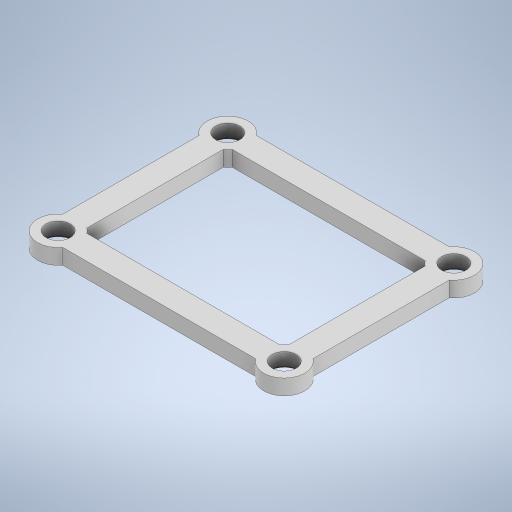
# Autodesk Inventor part: BasePlate
Saved by Autodesk Inventor 2024.2 (Build 282272000, 272)
## iProperties
Created: 2024-04-02
Part Number: BasePlate
Material: Generic
Document SubType Name: Modeling
Designer: ringl
Density: 1 g/cm^3
Appearance: Default
Author: ringl
Autodesk Inventor part; units mm, degrees
ref_plane "YZ Plane" through (0, 0, 0) normal (1, 0, 0) x (0, 1, 0)
ref_plane "XZ Plane" through (0, 0, 0) normal (0, 1, 0) x (-1, 0, 0)
ref_plane "XY Plane" through (0, 0, 0) normal (0, 0, 1) x (1, 0, 0)
sketch "Sketch1" plane through (0, 0, 0) normal (0, 1, 0) x (-1, 0, 0)
  circle A0 centre (0, 0) radius 2.35
  circle A1 centre (-44, 0) radius 2.35
  circle A2 centre (0, 33) radius 2.35
  circle A3 centre (-44, 33) radius 2.35
  line L0 (-3.2369, 30.65) -> (-40.7631, 30.65)
  line L1 (-40.7631, 35.35) -> (-3.2369, 35.35)
  line L2 (2.35, 29.7631) -> (2.35, 3.2369)
  line L3 (-2.35, 3.2369) -> (-2.35, 29.7631)
  line L4 (-3.2369, -2.35) -> (-40.7631, -2.35)
  line L5 (-40.7631, 2.35) -> (-3.2369, 2.35)
  arc A4 (-3.2369, -2.35) -> (2.35, 3.2369) centre (0, 0) ccw
  arc A5 (-2.35, 3.2369) -> (-3.2369, 2.35) centre (0, 0) ccw
  arc A6 (2.35, 29.7631) -> (-3.2369, 35.35) centre (0, 33) ccw
  arc A7 (-3.2369, 30.65) -> (-2.35, 29.7631) centre (0, 33) ccw
  line L6 (-41.65, 3.2369) -> (-41.65, 29.7631)
  line L7 (-46.35, 29.7631) -> (-46.35, 3.2369)
  arc A8 (-40.7631, 35.35) -> (-46.35, 29.7631) centre (-44, 33) ccw
  arc A9 (-41.65, 29.7631) -> (-40.7631, 30.65) centre (-44, 33) ccw
  arc A10 (-46.35, 3.2369) -> (-40.7631, -2.35) centre (-44, 0) ccw
  arc A11 (-40.7631, 2.35) -> (-41.65, 3.2369) centre (-44, 0) ccw
  dimension "d0" = 4.7
  dimension "d2" = 4.7
  dimension "d4" = 4.7
  dimension "d6" = 4.7
  dimension "d8" = 4
  dimension "d9" = 4
  dimension "d10" = 4
  dimension "d11" = 4
  dimension "d12" = 4
  dimension "d13" = 4
  dimension "d14" = 4
  dimension "d15" = 4
  dimension "d16" = 33
  dimension "d17" = 4.7
  dimension "d18" = 4.7
  dimension "d19" = 4.7
  dimension "d20" = 4.7
  dimension "d21" = 2.35
  dimension "d22" = 2.35
  dimension "d23" = 2.35
  dimension "d24" = 2.35
  dimension "d25" = 44
  constraints: 16 end point, 16 point on circle, 12 centre point, 5 coincident, 4 parallel, 2 horizontal, 2 horizontal alignment, 2 vertical alignment, 1 perpendicular, 1 vertical
  measures "d0" diameter of A0
  measures "d2" diameter of A1
  measures "d4" diameter of A2
  measures "d6" diameter of A3
  measures "d8" radius of A8
  measures "d9" radius of A6
  measures "d10" radius of A4
  measures "d11" radius of A10
  measures "d12" radius of A11
  measures "d13" radius of A9
  measures "d14" radius of A7
  measures "d15" radius of A5
  measures "d16" distance of A2.centre point (0, 0)
  measures "d17" distance between parallel lines of L1 L0
  measures "d18" distance between parallel lines of L7 L6
  measures "d19" distance between parallel lines of L4 L5
  measures "d20" distance between parallel lines of L2 L3
  measures "d21" distance from line of L0 A2.centre
  measures "d22" distance from line of A2.centre L3
  measures "d23" distance from line of L6 A3.centre
  measures "d24" distance from line of A1.centre L5
  measures "d25" distance of A1.centre point (0, 0)
extrude "Extrusion1" add sketch "Sketch1" along normal blind 3
chamfer "Chamfer1" distance 0.5 angle 45 4 edges at (2.35, 0, 33) (46.35, 0, 33) (46.35, 0, 0) (2.35, 0, 0)
body "Solid1"
